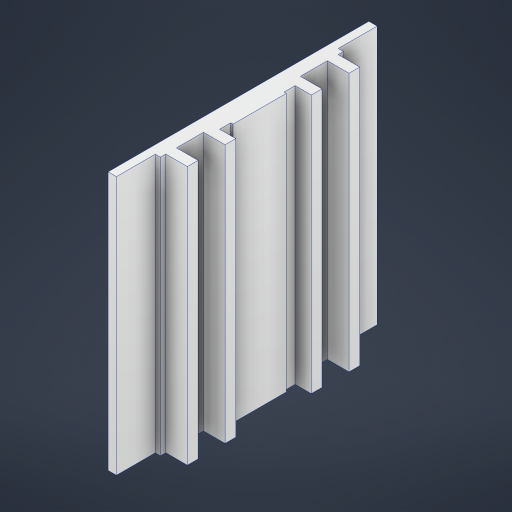
# Autodesk Inventor part: XmotorKreplenie
Saved by Autodesk Inventor 2024 (Build 280153000, 153)
## iProperties
Created: 2023-12-02
Part Number: XmotorKreplenie
Material: Aluminum 6061
Document SubType Name: Modeling
Designer: KirikDK
Mass: 2557.98 g
Surface Area: 1670.93 cm^2
Volume: 947.398 cm^3
Density: 2.7 g/cm^3
Appearance: Aluminum - Flat
Author: KirikDK
Autodesk Inventor part; units mm, degrees
ref_plane "YZ Plane" through (0, 0, 0) normal (1, 0, 0) x (0, 1, 0)
ref_plane "XZ Plane" through (0, 0, 0) normal (0, 1, 0) x (-1, 0, 0)
ref_plane "XY Plane" through (0, 0, 0) normal (0, 0, 1) x (1, 0, 0)
sketch "Sketch1" plane through (0, 0, 0) normal (0, 1, 0) x (-1, 0, 0)
  line L0 (15.8201, 44.4) -> (11, 44.4)
  line L1 (11, 39.4) -> (11, 39.4)
  line L2 (6, -15.8) -> (3.9, -15.8)
  line L3 (3.9, -15.8) -> (3.9, -40.6)
  line L4 (15.8201, 44.4) -> (15.8201, 80.4)
  line L5 (15.8201, 80.4) -> (23.5635, 80.4)
  line L6 (23.5635, 80.4) -> (23.5635, -40.6)
  line L7 (3.9, -40.6) -> (23.5635, -40.6)
  line L8 (6, -5.6) -> (-9, -5.6)
  line L9 (-9, -5.6) -> (-9, 4.4)
  line L10 (-9, 4.4) -> (11, 4.4)
  line L11 (11, 39.4) -> (-9, 39.4)
  line L12 (-9, 39.4) -> (-9, 29.4)
  line L13 (-9, 29.4) -> (11, 29.4)
  line L14 (6, -15.8) -> (6, -5.6)
  line L15 (11, 4.4) -> (11, 29.4)
  line L16 (11, 39.4) -> (11, 44.4)
  point P0 (0, 0)
  point P1 (6, 40.2)
  dimension "d3" = 5
  dimension "d8" = 10
  dimension "d9" = 36
  dimension "d13" = 45
  dimension "d14" = 24.8
  dimension "d15" = 10
  dimension "d17" = 5
  dimension "d18" = 2.1
  dimension "d19" = 10.2
  dimension "d21" = 35
  constraints: 34 end point, 5 perpendicular, 4 horizontal, 2 parallel, 2 vertical, 1 collinear
  measures "d3" distance of L0.end L1.start
  measures "d8" distance of L8.end L9.end
  measures "d9" distance of L0.start L4.end
  measures "d13" distance between parallel lines of L8 L1
  measures "d14" distance of L2.end L3.end
  measures "d15" distance of L11.end L12.end
  measures "d17" distance between parallel lines of L14 L16
  measures "d18" distance between parallel lines of L14 L3
  measures "d19" distance of L2.start L8.start
  measures "d21" distance from line of L3.end L8
extrude "Extrusion1" add sketch "Sketch1" along normal blind 240
mirror "Mirror1" about plane through (-3.9, 0, -40.6) normal (0, 0, -1) of "Extrusion1"
body "Solid1"
